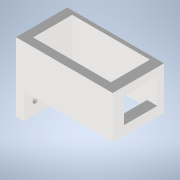
# Autodesk Inventor part: Part2
Saved by Autodesk Inventor 2021 (Build 250183000, 183)
## iProperties
Created: 2021-02-05
Part Number: Part2
Material: Generic
Document SubType Name: Modeling
Designer: Yuvraj Sandhu
Density: 1 g/cm^3
Appearance: Default
Author: Yuvraj Sandhu
Autodesk Inventor part; units mm, degrees
ref_plane "YZ Plane" through (0, 0, 0) normal (1, 0, 0) x (0, 1, 0)
ref_plane "XZ Plane" through (0, 0, 0) normal (0, 1, 0) x (-1, 0, 0)
ref_plane "XY Plane" through (0, 0, 0) normal (0, 0, 1) x (1, 0, 0)
sketch "Sketch1" plane through (0, 0, 0) normal (1, 0, 0) x (0, 1, 0)
  line L0 (0, 0) -> (-21.59, 0)
  line L1 (-21.59, 0) -> (-21.59, -29.21)
  line L2 (-21.59, -29.21) -> (0, -29.21)
  line L3 (0, -29.21) -> (0, 0)
  dimension "d25" = 29.21
  dimension "d26" = 21.59
  constraints: 8 end point, 2 parallel, 1 horizontal, 1 perpendicular
  measures "d25" distance of L0.end L1.end
  measures "d26" distance of L0.start L0.end
extrude "Extrusion1" add sketch "Sketch1" along normal blind 55
sketch "Sketch3" plane through (0, 0, 0) normal (0, 1, 0) x (1, 0, 0)
  line L0 (55, 26.9875) -> (5, 26.9875) projected
  line L1 (55, 4.7625) -> (5, 4.7625) projected
  line L2 (49.2125, 26.9875) -> (5, 26.9875)
  line L3 (5, 26.9875) -> (5, 4.7625)
  line L4 (5, 4.7625) -> (49.2125, 4.7625)
  line L5 (49.2125, 4.7625) -> (49.2125, 26.9875)
  point P0 (0, 0)
  constraints: 8 end point, 2 parallel, 1 horizontal, 1 perpendicular, 1 point on line
extrude "Extrusion3" cut sketch "Sketch3" against normal blind 25
sketch "Sketch4" plane through (55, 0, 0) normal (1, 0, 0) x (0, 0, -1)
  line L0 (25.4, -19.05) -> (6.35, -19.05)
  line L1 (6.35, -19.05) -> (6.35, -4.7625)
  line L2 (6.35, -4.7625) -> (25.4, -4.7625)
  line L3 (25.4, -4.7625) -> (25.4, -19.05)
  point P0 (0, 0)
  constraints: 8 end point, 2 parallel, 1 horizontal, 1 perpendicular
extrude "Extrusion4" cut sketch "Sketch4" against normal blind 25
body "Solid1"
